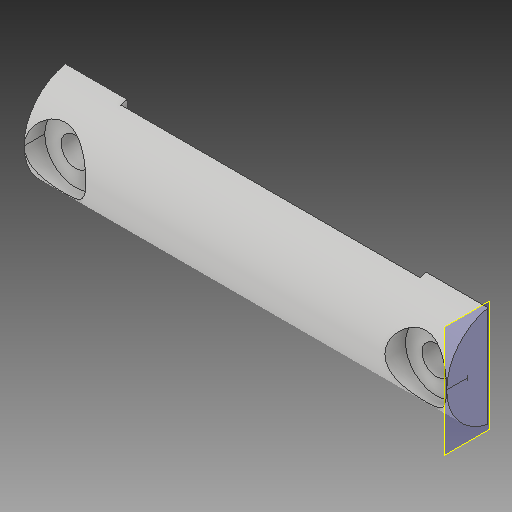
# Autodesk Inventor part: SR-T-09
Saved by Autodesk Inventor 2019.4 (Build 234330000, 330)
## iProperties
Created: 2019-07-23
Part Number: SR-T-09
Material: 一般
Document SubType Name: Modeling
Designer: Koki Shinjo
Mass: 0.113783 g
Surface Area: 2.63143 cm^2
Volume: 0.113783 cm^3
Density: 1 g/cm^3
Appearance: 既定
Author: Koki Shinjo
Autodesk Inventor part; units mm, degrees
ref_plane "作業平面1" through (15, -6, 0) normal (-1, 0, 0) x (0, -1, 0)
sketch "スケッチ1" plane through (15, -6, 0) normal (-1, 0, 0) x (0, -1, 0)
  arc A0 (-0.0505, 0) -> (-4.9495, 0) centre (-2.5, -0.5) ccw projected
  line L0 (-4.9495, 0) -> (-0.0505, 0) projected
  point P0 (-6, 0)
ref_plane "作業平面2" through (-5.5, -5.9495, 0) normal (1, 0, 0) x (0, 1, 0)
extrude "押し出し1" add sketch "スケッチ1" along normal up to surface (20.5 mm away)
ref_plane "作業平面3" through (12, 0, -1) normal (0, 0, -1) x (-1, 0, 0)
sketch "スケッチ2" plane through (12, 0, 0) normal (0, 0, -1) x (-1, 0, 0)
  line L0 (14.5, -5.9495) -> (17.5, -5.9495) construction
  line L1 (14.5, -1.0505) -> (14.5, -5.9495) construction
  line L2 (17.5, -1.0505) -> (14.5, -1.0505) construction
  line L3 (17.5, -5.9495) -> (17.5, -1.0505) construction
  arc A0 (0, -3) -> (0.5, -3.5) centre (0.5, -3) ccw construction
  line L4 (0.5, -3.5) -> (7.401, -3.5) construction
  arc A1 (7.401, -3.5) -> (7.901, -3) centre (7.401, -3) ccw construction
  line L5 (7.901, -3) -> (7.901, -2.5) construction
  arc A2 (7.901, -2.5) -> (7.401, -2) centre (7.401, -2.5) ccw construction
  line L6 (7.401, -2) -> (0.5, -2) construction
  arc A3 (0.5, -2) -> (0, -2.5) centre (0.5, -2.5) ccw construction
  line L7 (0, -3) -> (0, -2.5) construction
  spline S0 degree 3 poles (8.201, -0.8167) (8.2004, -0.8173) (8.1998, -0.8179) (8.1567, -0.8609) (8.1131, -0.8989) (8.0137, -0.9678) (7.9594, -0.997) (7.8435, -1.0385) (7.7825, -1.0505) (7.721, -1.0505) knots -0.000247 -0.000247 -0.000247 -0.000247 0 0 0.018039 0.018039 0.036793 0.036793 0.055658 0.055658 0.055658 0.055658 construction
  line L8 (8.201, -0.3) -> (8.201, -0.8167) construction
  line L9 (11.7, -0.3) -> (8.201, -0.3) construction
  line L10 (11.7, -4.5) -> (11.7, -0.3) construction
  line L11 (11.7, -4.5) -> (0.3, -4.5) construction
  arc A4 (0.3, -4.5) -> (0, -4.8) centre (0.3, -4.8) ccw construction
  line L12 (0, -5.9495) -> (0, -4.8) construction
  line L13 (-3, -5.9495) -> (0, -5.9495) construction
  line L14 (-3, -1.0505) -> (-3, -5.9495) construction
  line L15 (7.721, -1.0505) -> (-3, -1.0505) construction
  line L16 (17.5, -1.0505) -> (17.5, -5.9495) construction
  line L17 (-3, -1.0505) -> (17.5, -1.0505) construction
  line L18 (-3, -5.9495) -> (-3, -1.0505) construction
  line L19 (-3, -5.9495) -> (17.5, -5.9495) construction
  line L20 (14.5, -5.9495) -> (0, -5.9495)
  line L21 (0, -5.9495) -> (0, -1.0505)
  line L22 (0, -1.0505) -> (14.5, -1.0505)
  line L23 (14.5, -1.0505) -> (14.5, -5.9495)
  circle A5 centre (16, -3.5) radius 0.55 projected
  circle A6 centre (-1.5, -3.5) radius 0.55 projected
  point P0 (12, 0)
  constraints: 8 end point, 2 parallel, 2 point on line, 1 horizontal, 1 perpendicular
extrude "押し出し2" cut sketch "スケッチ2" against normal blind 0.3 contours L20 L21 L22 L23
sketch "スケッチ3" plane through (15, -5.9495, 0) normal (0, 0, -1) x (-1, 0, 0)
  line L0 (17.5, 4.899) -> (17.5, 0) construction
  line L1 (17.5, 0) -> (20.5, 0) construction
  line L2 (20.5, 4.899) -> (20.5, 0) construction
  line L3 (17.5, 4.899) -> (20.5, 4.899) construction
  line L4 (3, 0) -> (3, 4.899) construction
  line L5 (0, 4.899) -> (3, 4.899) construction
  line L6 (0, 0) -> (0, 4.899) construction
  line L7 (0, 0) -> (3, 0) construction
  line L8 (20.5, 0) -> (20.5, 4.899) construction
  line L9 (20.5, 0) -> (17.5, 4.899) construction
  line L10 (17.5, 0) -> (20.5, 0) construction
  line L11 (17.5, 0) -> (20.5, 4.899) construction
  line L12 (0, 0) -> (0, 4.899) construction
  line L13 (3, 4.899) -> (0, 0) construction
  line L14 (0, 4.899) -> (3, 4.899) construction
  line L15 (0, 0) -> (0, 4.899) construction
  line L16 (3, 0) -> (3, 4.899) construction
  line L17 (0, 4.899) -> (3, 0) construction
  circle A0 centre (19, 2.4495) radius 0.7
  circle A1 centre (1.5, 2.4495) radius 0.7
  point P0 (15, 5.9495)
  dimension "d5" = 1.4
  constraints: 10 end point, 3 equal length, 2 centre point, 2 midpoint, 1 equal radius
  measures "d5" diameter of A1
extrude "押し出し3" cut sketch "スケッチ3" against normal up to next
ref_plane "作業平面5" through (15, -3.5, 1) normal (0, 0, -1) x (-1, 0, 0)
ref_plane "作業平面4" through (15, -3.5, 2) normal (0, 0, -1) x (-1, 0, 0)
sketch "スケッチ4" plane through (15, -3.5, 2) normal (0, 0, -1) x (-1, 0, 0)
  circle A0 centre (19, 0) radius 1.5
  circle A1 centre (1.5, 0) radius 0.7 projected
  circle A2 centre (1.5, 0) radius 1.5
  circle A3 centre (19, 0) radius 0.7 projected
  point P0 (15, 3.5)
  point P1 (19, 0.7)
  point P2 (1.5, 0.7)
  dimension "d9" = 3
  constraints: 2 centre point, 2 vertical alignment, 1 coincident, 1 equal radius, 3 other
  measures "d9" diameter of A2
extrude "押し出し4" cut sketch "スケッチ4" along normal up to surface (1 mm away) contours A0 | A1 | A2 | A3
